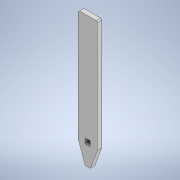
# Autodesk Inventor part: graduated_foot_03
Saved by Autodesk Inventor 2020 (Build 240168000, 168)
## iProperties
Created: 2019-12-19
Part Number: graduated_foot_03
Material: Générique
Document SubType Name: Modeling
Designer: damien
Density: 1 g/cm^3
Appearance: Par défaut
Author: damien
Autodesk Inventor part; units mm, degrees
ref_plane "YZ Plane" through (0, 0, 0) normal (1, 0, 0) x (0, 1, 0)
ref_plane "XZ Plane" through (0, 0, 0) normal (0, 1, 0) x (-1, 0, 0)
ref_plane "XY Plane" through (0, 0, 0) normal (0, 0, 1) x (1, 0, 0)
sketch "Esquisse1" plane through (0, 0, 0) normal (0, 0, 1) x (1, 0, 0)
  line L0 (0, 0) -> (80, 0)
  line L1 (80, 0) -> (80, 550)
  line L2 (80, 550) -> (0, 550)
  line L3 (0, 550) -> (0, 0)
  dimension "d0" = 80
  dimension "d1" = 550
  constraints: 8 end point, 2 parallel, 1 horizontal, 1 perpendicular
  measures "d0" distance of L0.start L0.end
  measures "d1" distance of L2.end L0.start
extrude "Extrusion1" add sketch "Esquisse1" along normal blind 18.55
chamfer "Chanfrein1" distance 5 angle 45 2 edges at (0, 550, 9.275) (80, 550, 9.275)
sketch "Esquisse4" plane through (0, 0, 18.55) normal (0, 0, 1) x (1, 0, 0)
  line L0 (0, 545) -> (0, 0) projected
  line L1 (80, 0) -> (80, 545) projected
  line L2 (0, 80) -> (29.1176, 0)
  line L3 (0, 0) -> (80, 0) projected
  line L4 (50.8824, 0) -> (80, 80)
  line L5 (29.1176, 0) -> (50.8824, 0)
  line L6 (30, 100) -> (50, 100)
  line L7 (50, 100) -> (50, 80)
  line L8 (50, 80) -> (30, 80)
  line L9 (30, 80) -> (30, 100)
  line L10 (40, 0) -> (40, 80) construction
  dimension "d23" = 70
  dimension "d24" = 70
  dimension "d25" = 80
  dimension "d26" = 20
  dimension "d27" = 20
  constraints: 16 end point, 5 point on line, 2 midpoint, 2 parallel, 1 collinear, 1 equal length, 1 horizontal, 1 perpendicular, 1 vertical
  measures "d23" angle of L3 L2
  measures "d24" angle of L3 L4
  measures "d25" distance from line of L3 L2.start
  measures "d26" distance of L7.end L8.end
  measures "d27" distance of L6.end L7.end
extrude "Extrusion3" cut sketch "Esquisse4" against normal blind 20
